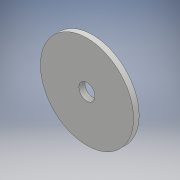
# Autodesk Inventor part: 071_0204_RollCutter20mmScrewClamp8mm
Saved by Autodesk Inventor 2018 (Build 220112000, 112)
## iProperties
Created: 2018-07-06
Part Number: 071_0204_RollCutter20mmScrewClamp8mm
Material: Generic
Document SubType Name: Modeling
Designer: deniz
Density: 1 g/cm^3
Appearance: Default
Author: deniz
Autodesk Inventor part; units mm, degrees
ref_plane "YZ Plane" through (0, 0, 0) normal (1, 0, 0) x (0, 1, 0)
ref_plane "XZ Plane" through (0, 0, 0) normal (0, 1, 0) x (-1, 0, 0)
ref_plane "XY Plane" through (0, 0, 0) normal (0, 0, 1) x (1, 0, 0)
sketch "Sketch1" plane through (0, 0, 0) normal (0, 1, 0) x (-1, 0, 0)
  circle A0 centre (0, 0) radius 2.6
  circle A1 centre (0, 0) radius 4
  circle A2 centre (0, 0) radius 15
  circle A3 centre (0, 0) radius 13
  dimension "d21" = 5.2
  dimension "d22" = 8
  dimension "d23" = 30
  dimension "d31" = 2
  constraints: 4 centre point, 4 coincident
  measures "d21" diameter of A0
  measures "d22" diameter of A1
  measures "d23" diameter of A2
  measures "d31" radial gap between concentric circles of A2 A3
extrude "Extrusion6" add sketch "Sketch1" against normal blind 1.5 contours A1 | A2 | A3
extrude "Extrusion7" add sketch "Sketch1" along normal blind 0.45 contours A1
chamfer "Chamfer1" distance 0.25 angle 60 1 edges at (4, 0, 0) measured on face at (-11.188, 0, -1.1966)
extrude "Extrusion8" add sketch "Sketch1" along normal blind 0.3 contours A2
body "Solid3"
